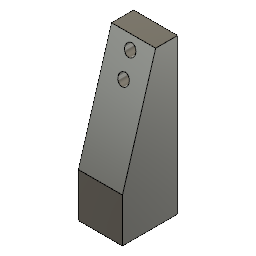
sphinx mod v11 (Autodesk Fusion 360 archive; units mm, degrees)
design "2040base"
Autodesk Fusion 360 part; units mm, degrees
sketch "Sketch1" plane through (0, 0, 0) normal (0, 0, 1) x (1, 0, 0)
  line L0 (0, 0) -> (40, 0)
  line L1 (40, 0) -> (40, 140)
  line L2 (40, 140) -> (0, 140)
  line L3 (0, 140) -> (0, 0)
  circle A0 centre (20, 130) radius 2.75
  circle A1 centre (20, 110) radius 2.75
  dimension "d1" = 40
  dimension "d2" = 140
  dimension "d3" = 5.5
  dimension "d4" = 20
  dimension "d5" = 10
  dimension "d6" = 5.5
  dimension "d7" = 20
  dimension "d8" = 20
  measures "d3" diameter of A0
  measures "d6" diameter of A1
extrude "Extrude1" add sketch "Sketch1" along normal blind 50
hole "Hole1" at (20, 130, 50) direction (0, 0, -1) diameter 10 depth 35 tip angle 180
hole "Hole2" at (20, 110, 50) direction (0, 0, -1) diameter 10 depth 35 tip angle 180
sketch "Sketch2" plane through (40, 0, 0) normal (1, 0, 0) x (0, 0, -1)
  line L0 (0, 0) -> (0, 140)
  line L1 (0, 140) -> (-50, 140)
  line L2 (-50, 140) -> (-50, 0)
  line L3 (-50, 0) -> (0, 0)
  line L4 (-50, 140) -> (-20, 140)
  line L5 (-50, 140) -> (-50, 40)
  line L6 (-50, 40) -> (-20, 140)
extrude "Extrude2" cut sketch "Sketch2" against normal blind 40 contours L1 L2 L4 L5 L6
